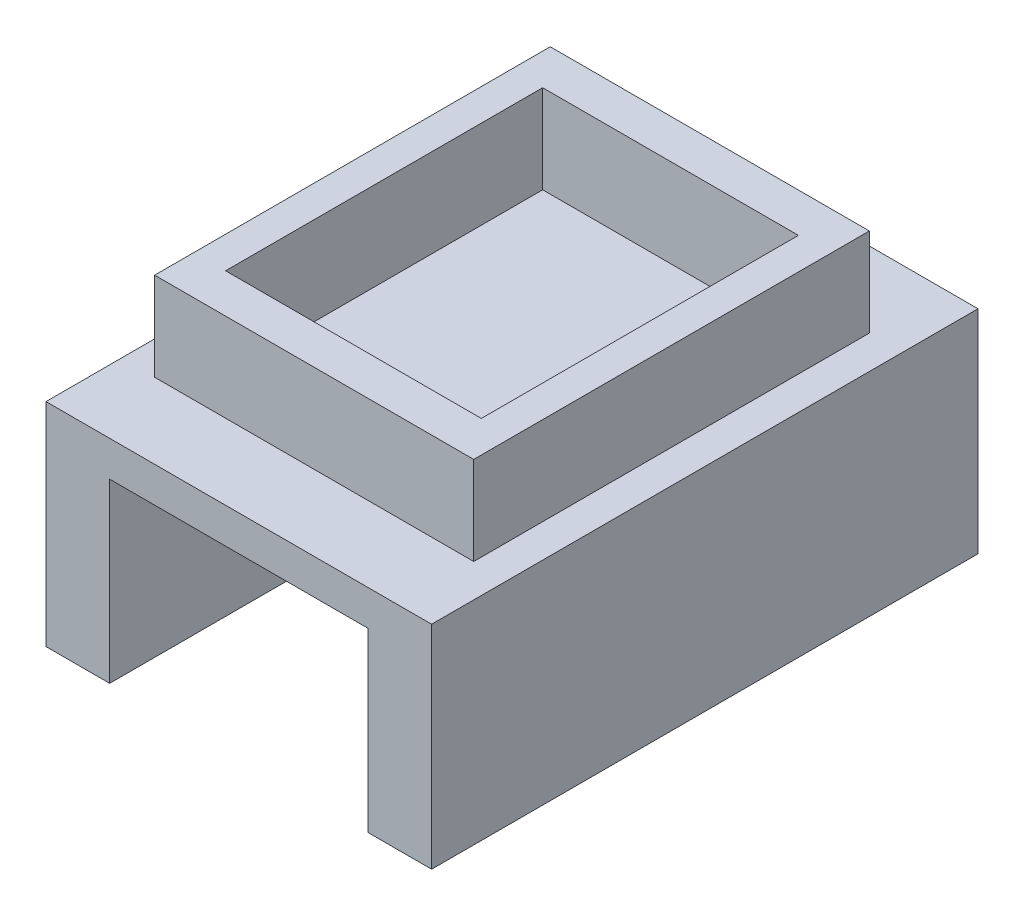
# Autodesk Inventor part: Lead_Screw_Motor_Mount
Saved by Autodesk Inventor 2015 (Build 190159000, 159)
## iProperties
Created: 2014-12-28
Part Number: Lead_Screw_Motor_Mount
Material: Generic
Document SubType Name: Modeling
Designer: Drew
Density: 1 g/cm^3
Appearance: Default
Author: Drew
Autodesk Inventor part; units mm, degrees
ref_plane "YZ Plane" through (0, 0, 0) normal (1, 0, 0) x (0, 1, 0)
ref_plane "XZ Plane" through (0, 0, 0) normal (0, 1, 0) x (-1, 0, 0)
ref_plane "XY Plane" through (0, 0, 0) normal (0, 0, 1) x (1, 0, 0)
sketch "Sketch1" plane through (0, 0, 0) normal (0, 1, 0) x (-1, 0, 0)
  line L0 (-11.4576, -14.2058) -> (11.4576, -14.2058)
  line L1 (11.4576, -14.2058) -> (11.4576, 14.2058)
  line L2 (11.4576, 14.2058) -> (-11.4576, 14.2058)
  line L3 (-11.4576, 14.2058) -> (-11.4576, -14.2058)
  line L4 (-11.4576, -14.2058) -> (11.4576, 14.2058) construction
  line L5 (11.4576, -14.2058) -> (-11.4576, 14.2058) construction
  line L6 (-9.1832, -11.3858) -> (9.1832, -11.3858)
  line L7 (9.1832, -11.3858) -> (9.1832, 11.3858)
  line L8 (9.1832, 11.3858) -> (-9.1832, 11.3858)
  line L9 (-9.1832, 11.3858) -> (-9.1832, -11.3858)
  line L10 (-9.1832, -11.3858) -> (9.1832, 11.3858) construction
  line L11 (9.1832, -11.3858) -> (-9.1832, 11.3858) construction
  point P0 (0, 0)
  constraints: 24 end point, 4 midpoint, 4 parallel, 2 horizontal, 2 perpendicular, 1 point on line
extrude "Extrusion1" add sketch "Sketch1" along normal blind 6.35
sketch "Sketch2" plane through (0, 0, 0) normal (0, -1, 0) x (1, 0, 0)
  line L0 (-13.8467, -19.6194) -> (13.8467, -19.6194)
  line L1 (13.8467, -19.6194) -> (13.8467, 19.6194)
  line L2 (13.8467, 19.6194) -> (-13.8467, 19.6194)
  line L3 (-13.8467, 19.6194) -> (-13.8467, -19.6194)
  line L4 (-13.8467, -19.6194) -> (13.8467, 19.6194) construction
  line L5 (13.8467, -19.6194) -> (-13.8467, 19.6194) construction
  point P0 (0, 0)
  constraints: 12 end point, 2 midpoint, 2 parallel, 1 horizontal, 1 perpendicular
extrude "Extrusion2" add sketch "Sketch2" along normal blind 2.54
sketch "Sketch3" plane through (0, -2.54, 0) normal (0, -1, 0) x (1, 0, 0)
  line L0 (-13.8467, -19.6194) -> (13.8467, -19.6194) projected
  line L1 (13.8467, 19.6194) -> (9.2756, 19.6194)
  line L2 (9.2756, 19.6194) -> (9.2756, -19.6194)
  line L3 (9.2756, -19.6194) -> (13.8467, -19.6194)
  line L4 (13.8467, -19.6194) -> (13.8467, 19.6194)
  line L5 (0, 28.8749) -> (0, -37.3644)
  line L6 (-13.8467, 19.6194) -> (-9.2756, 19.6194)
  line L7 (-9.2756, 19.6194) -> (-9.2756, -19.6194)
  line L8 (-9.2756, -19.6194) -> (-13.8467, -19.6194)
  line L9 (-13.8467, -19.6194) -> (-13.8467, 19.6194)
  point P0 (0, 0)
  constraints: 18 end point, 5 symmetric about line, 2 parallel, 1 horizontal, 1 perpendicular, 1 point on line, 1 vertical
extrude "Extrusion3" add sketch "Sketch3" along normal blind 12.7
body "Solid1"
